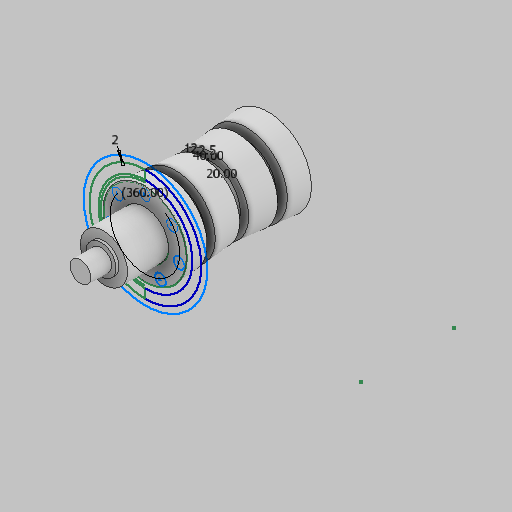
# Autodesk Inventor part: vall
Saved by Autodesk Inventor 2026 (Build 300175000, 175)
## iProperties
Created: 2026-07-30
Part Number: vall
Material: Типовые
Document SubType Name: Modeling
Designer: admin
Density: 1 g/cm^3
Appearance: По умолчанию
Author: admin
Autodesk Inventor part; units mm, degrees
ref_plane "YZ Plane" through (0, 0, 0) normal (1, 0, 0) x (0, 1, 0)
ref_plane "РабПлоскость1" through (-73.278894, 6.789202, 50.733011) normal (1, 0, 0) x (0, 1, 0)
sketch "Эскиз1" plane through (-73.278894, 6.789202, 50.733011) normal (1, 0, 0) x (0, 1, 0)
  line L0 (-58.5, -54.576442) -> (-56.806889, -56.269553)
  line L1 (-56.806889, -56.269553) -> (-56.806889, -58.269553)
  line L2 (-56.806889, -58.269553) -> (-58.5, -58.269553)
  line L3 (-58.5, -58.269553) -> (-58.5, -84.609012)
  line L4 (-58.5, -84.609012) -> (-61.5, -84.609012)
  line L5 (-61.5, -84.609012) -> (-61.5, -36)
  line L6 (-61.5, -36) -> (-58.5, -36)
  line L7 (-58.5, -36) -> (-58.5, -54.576442)
  circle A0 centre (-40.306889, -36) radius 26
  line L8 (7.025, 0) -> (-7.025, 0)
  line L9 (0.754403, -80) -> (0, 0)
  line L10 (-17.048737, -57.000934) -> (-15.211393, -36)
  line L11 (-15.211393, -36) -> (-17.048737, -14.999066)
  line L12 (-17.048737, -14.999066) -> (0.139913, -14.836977)
  line L13 (-17.048737, -57.000934) -> (0.535957, -56.835109)
  line L14 (-7.463687, -56.910546) -> (-7.990926, -1)
  line L15 (-3.59101, 0) -> (-3.59101, 7)
  line L16 (-3.59101, 7) -> (-0.06601, 7)
  line L17 (-0.06601, 7) -> (0, 0)
  line L18 (-2.035648, -57) -> (-3.035648, -57)
  line L19 (-3.035648, -57) -> (-3.006712, -60.068517)
  line L20 (-2.035648, -57) -> (-2.035648, -45)
  line L21 (-2.035648, -45) -> (0.424352, -45)
  line L22 (-7.990926, -1) -> (-5.09101, -1)
  line L23 (-5.09101, -1) -> (-5.09101, 0)
  line L24 (-7.463687, -56.910546) -> (-7.463687, -60.110546)
  line L25 (-7.463687, -60.110546) -> (0.566131, -60.034825)
  circle A1 centre (-40.306889, -36) radius 25
  line L26 (-14.03976, -14.970692) -> (-12.199934, -36)
  line L27 (-12.199934, -36) -> (-14.034791, -56.972512)
  ellipse E0 centre (0.583116, -80.125072) end of major axis (5.383116, -80.1252) minor radius 0.032213
  point P0 (-6.789202, -50.733011)
  point P1 (-3.46, -57)
  dimension "d0" = 170
  dimension "d1" = 42
  dimension "d6" = 7
  dimension "d8" = 8
  dimension "d10" = 12
  dimension "d11" = 3.525
  dimension "d12" = 1.5
  dimension "d13" = 1
  dimension "d14" = 2.46
  dimension "d15" = 1
  dimension "d58" = 3.2
  dimension "d66" = 1
  dimension "d70" = 3
  constraints: 54 end point, 9 point on line, 8 perpendicular, 6 horizontal, 6 vertical, 2 centre point, 2 horizontal alignment, 2 parallel, 2 tangent, 1 coincident, 1 collinear, 1 equal length, 1 midpoint, 12 other
  measures "d0" angle of L11 L10
  measures "d1" distance between parallel lines of L12 L13
  measures "d6" distance between parallel lines of L16 L8
  measures "d8" distance between parallel lines of L9 L14
  measures "d10" distance of L18.start L20.end
  measures "d11" distance of L15.end L16.end
  measures "d12" distance between parallel lines of L15 L23
  measures "d13" distance of L22.end L23.end
  measures "d14" distance of L20.end L21.end
  measures "d15" distance of L18.start L18.end
  measures "d58" distance of L14.start L24.end
  measures "d66" radial gap between concentric circles of A0 A1
  measures "d70" distance between parallel lines of L11 L26
sketch "Эскиз1 outline for Вращение1" plane through (-73.278894, 6.789202, 50.733011) normal (1, 0, 0) x (0, 1, 0)
  line L0 (-17.048737, -57.000934) -> (0.535957, -56.835109)
  line L1 (-15.211393, -36) -> (-17.048737, -57.000934)
  line L2 (-17.048737, -14.999066) -> (-15.211393, -36)
  line L3 (0.139913, -14.836977) -> (-17.048737, -14.999066)
  line L4 (0.535957, -56.835109) -> (0.139913, -14.836977)
revolve "Вращение1" add sketch "Эскиз1 outline for Вращение1" angle 360 about axis through (-73.278894, 7.543605, -29.266989) along (0, -0.0094296, 0.9999555)
sketch "Эскиз2" plane through (-73.278894, 6.789202, 50.733011) normal (1, 0, 0) x (0, 1, 0)
  line L0 (0.754403, -80) -> (0, 0)
  line L1 (-0.06601, 7) -> (0, 0)
  line L2 (-3.59101, 7) -> (-0.06601, 7)
  line L3 (-3.59101, 0) -> (-3.59101, 7)
  line L4 (7.025, 0) -> (-7.025, 0)
  line L5 (-5.09101, -1) -> (-5.09101, 0)
  line L6 (-7.990926, -1) -> (-5.09101, -1)
  line L7 (-7.463687, -56.910546) -> (-7.990926, -1)
  line L8 (-17.048737, -57.000934) -> (0.535957, -56.835109)
  line L9 (-3.035648, -57) -> (-3.006712, -60.068517)
  line L10 (-2.035648, -57) -> (-2.035648, -45)
  line L11 (-2.035648, -57) -> (-3.035648, -57)
  line L12 (-2.035648, -45) -> (0.424352, -45)
  line L13 (-13.118565, -46.5) -> (-9.5, -46.5)
  line L14 (-9.5, -46.5) -> (-9.5, -49.5)
  line L15 (-9.5, -49.5) -> (-13.381031, -49.5)
  line L16 (-7.463687, -60.110546) -> (0.566131, -60.034825)
  line L17 (-7.463687, -56.910546) -> (-7.463687, -60.110546)
  line L18 (-14.03976, -14.970692) -> (-12.199934, -36)
  line L19 (-12.199934, -36) -> (-14.034791, -56.972512)
  line L20 (-14.03976, -14.970692) -> (-7.859731, -14.912414)
  line L21 (-12.199934, -36) -> (-8, -36) construction
  line L22 (-9.5, -36) -> (-9.5, -37.5)
  line L23 (-9.5, -37.5) -> (-12.331167, -37.5)
  line L24 (-13.118565, -25.5) -> (-9.5, -25.5)
  line L25 (-9.5, -25.5) -> (-9.5, -22.5)
  line L26 (-9.5, -22.5) -> (-13.381031, -22.5)
  line L27 (-9.5, -36) -> (-9.5, -34.5)
  line L28 (-9.5, -34.5) -> (-12.331167, -34.5)
  point P0 (0.535957, -56.835109)
  point P1 (-3.46, -57)
  point P2 (-2.035648, -56.85936)
  dimension "d71" = 3
  dimension "d72" = 1.5
  dimension "d73" = 1.5
  constraints: 24 end point, 6 symmetric about line, 4 point on line, 3 horizontal, 2 perpendicular, 1 collinear, 1 vertical, 5 other
  measures "d71" distance of L13.end L14.end
  measures "d73" distance of L22.start L22.end
sketch "Эскиз2 outline for Вращение2" plane through (-73.278894, 6.789202, 50.733011) normal (1, 0, 0) x (0, 1, 0)
  line L0 (-9.5, -46.5) -> (-9.5, -49.5)
  line L1 (-9.5, -49.5) -> (-13.381031, -49.5)
  line L2 (-13.381031, -49.5) -> (-14.034791, -56.972512)
  line L3 (-14.034791, -56.972512) -> (-7.463687, -56.910546)
  line L4 (-7.463687, -56.910546) -> (-7.463687, -60.110546)
  line L5 (-7.463687, -60.110546) -> (0.566131, -60.034825)
  line L6 (0.566131, -60.034825) -> (-0.06601, 7)
  line L7 (-0.06601, 7) -> (-3.59101, 7)
  line L8 (-3.59101, 7) -> (-3.59101, 0)
  line L9 (-3.59101, 0) -> (-5.09101, 0)
  line L10 (-5.09101, 0) -> (-5.09101, -1)
  line L11 (-5.09101, -1) -> (-7.990926, -1)
  line L12 (-7.990926, -1) -> (-7.859731, -14.912414)
  line L13 (-7.859731, -14.912414) -> (-14.03976, -14.970692)
  line L14 (-14.03976, -14.970692) -> (-13.381031, -22.5)
  line L15 (-13.381031, -22.5) -> (-9.5, -22.5)
  line L16 (-9.5, -22.5) -> (-9.5, -25.5)
  line L17 (-9.5, -25.5) -> (-13.118565, -25.5)
  line L18 (-13.118565, -25.5) -> (-12.331167, -34.5)
  line L19 (-12.331167, -34.5) -> (-9.5, -34.5)
  line L20 (-9.5, -34.5) -> (-9.5, -37.5)
  line L21 (-9.5, -37.5) -> (-12.331167, -37.5)
  line L22 (-12.331167, -37.5) -> (-13.118565, -46.5)
  line L23 (-13.118565, -46.5) -> (-9.5, -46.5)
revolve "Вращение2" add sketch "Эскиз2 outline for Вращение2" angle 360 about axis through (-73.278894, 7.543605, -29.266989) along (0, -0.0094296, 0.9999555) separate body
sketch "Эскиз3" plane through (-73.406488, 6.789202, 4.233011) normal (0, 0, -1) x (-1, 0, 0)
  arc A0 (11.276311, -4.104242) -> (11.276311, 4.104242) centre (0, 0) ccw
  arc A1 (8.92708, -3.249191) -> (8.92708, 3.249191) centre (0, 0) ccw
  line L0 (8.92708, -3.249191) -> (11.276311, -4.104242)
  line L1 (8.92708, 3.249191) -> (11.276311, 4.104242)
  circle A2 centre (0, 0) radius 3.525 construction
  point P0 (-73.406488, -6.789202)
  point P1 (8, 0)
  dimension "d30" = 2.5
  dimension "d31" = 40
  dimension "d32" = 20
  dimension "d74" = 12
  constraints: 4 end point, 4 point on circle, 3 coincident, 2 centre point, 2 point on line, 1 horizontal alignment
  measures "d30" radial gap between concentric circles of A0 A1
  measures "d31" angle of L1 L0
  measures "d74" radius of A0
extrude "Выдавливание1" [suppressed]
pattern_circular "Круговой массив2" [suppressed]
fillet "Сопряжение1" radius 1 2 edges at (-73.2789, 24.1178, 36.0581) (-73.2789, 24.9099, -5.9363)
sketch "Эскиз4" plane through (-73.278894, 6.789202, 50.733011) normal (1, 0, 0) x (0, 1, 0)
  line L0 (17.019009, -56.679673) -> (-15.947094, -56.990545)
  line L1 (-15.967754, -14.988873) -> (16.24758, -14.685081)
  line L2 (-15.967754, -14.988873) -> (16.24758, -14.685081)
  line L3 (16.24758, -14.685081) -> (19.566131, -14.685081)
  line L4 (19.566131, -14.685081) -> (19.566131, -60.034825)
  line L5 (19.566131, -60.034825) -> (0.566131, -60.034825)
  line L6 (0, -60.034825) -> (0, -15)
  line L7 (-7.463687, -60.110546) -> (0.566131, -60.034825)
  point P0 (-6.789202, -50.733011)
  dimension "d40" = 19
  constraints: 6 end point, 1 horizontal, 1 perpendicular, 1 vertical, 5 other
  measures "d40" distance of L5.end L4.end
revolve "Вращение3" [suppressed]
feature "Комбинировать1" [suppressed]
ref_plane "РабПлоскость3" through (-73.278894, 23.808211, -5.946662) normal (0, 0.0094296, -0.9999555) x (-1, 0, 0)
feature "Разделение3" [suppressed]
feature "Разделение4" [suppressed]
sketch "Эскиз5" plane through (-73.406488, 6.789202, -6.266989) normal (0, 0, -1) x (-1, 0, 0)
  circle A0 centre (0, 0) radius 3.46
  circle A1 centre (0, 0) radius 2.46
  arc A2 (0, -19) -> (0, 19) centre (0, 0) ccw
  arc A3 (0, -15.211393) -> (0, 15.211393) centre (0, 0) ccw
  circle A4 centre (0, 0) radius 21
  arc A5 (0, 19) -> (0, -19) centre (0, 0) ccw
  point P0 (-73.406488, -6.789202)
  dimension "d42" = 2
  constraints: 2 centre point, 2 coincident, 2 point on circle
  measures "d42" radial gap between concentric circles of A4 A2
extrude "Выдавливание2" [suppressed]
sketch "Эскиз6" plane through (-73.406488, 6.789202, 35.733011) normal (0, 0, 1) x (1, 0, 0)
  line L0 (0, 19) -> (0, 15.957347)
  arc A0 (0, 15.957347) -> (0, -15.957347) centre (0, 0) ccw
  line L1 (0, -15.957347) -> (0, -19)
  arc A1 (0, 19) -> (0, -19) centre (0, 0) ccw
  circle A2 centre (0, 0) radius 8
  arc A3 (0, -15.957347) -> (0, 15.957347) centre (0, 0) ccw
  arc A4 (0, 15.211393) -> (0, -15.211393) centre (0, 0) ccw
  arc A5 (0, -19) -> (0, 19) centre (0, 0) ccw
  circle A6 centre (0, 0) radius 21
  circle A7 centre (0, 11.834908) radius 1.856866
  circle A8 centre (-9.252903, 7.378944) radius 1.856866
  circle A9 centre (-11.538182, -2.633515) radius 1.856866
  circle A10 centre (-5.134974, -10.662883) radius 1.856866
  circle A11 centre (5.134974, -10.662883) radius 1.856866
  circle A12 centre (11.538182, -2.633515) radius 1.856866
  circle A13 centre (9.252903, 7.378944) radius 1.856866
  circle A14 centre (0, 0) radius 14.037196
  circle A15 centre (0, 0) radius 8
  point P0 (73.406488, -6.789202)
  point P1 (-4.698463, -1.710101)
  point P2 (-1.710101, -4.698463)
  point P3 (0, 19)
  dimension "d45" = 2
  dimension "d64" = 360
  constraints: 10 centre point, 4 point on circle, 3 coincident, 15 other
  measures "d45" radial gap between concentric circles of A6 A1
extrude "Выдавливание3" [suppressed]
extrude "Выдавливание4" [suppressed]
extrude "Выдавливание6" [suppressed]
feature "Толщина1" [suppressed]
feature "Толщина2" [suppressed]
feature "Толщина3" [suppressed]
feature "Толщина4" [suppressed]
chamfer "Фаска1" distance 2 angle 45 1 edges at (-73.2789, 15.3852, -9.2261)
equation "\"d50\" = backflash"
equation "\"d79\" = backflash"
equation "\"d54\" = backflash"
equation "\"d80\" = backflash"
equation "\"backflash\" = 0.12"
